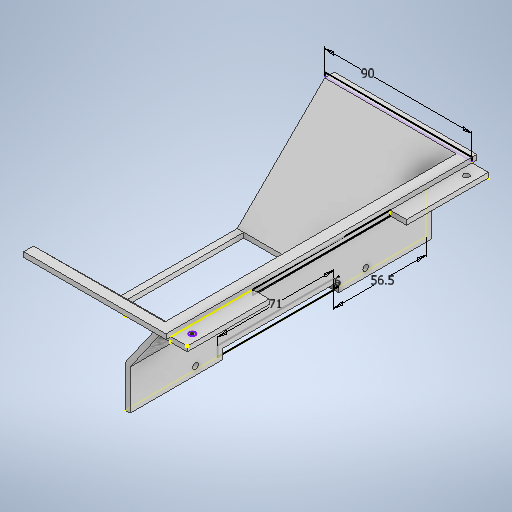
# Autodesk Inventor part: D2-CA
Saved by Autodesk Inventor 2025.2 (Build 292293000, 293)
## iProperties
Created: 2025-11-16
Part Number: D2-CA
Material: 일반
Document SubType Name: Modeling
Designer: RunGeun
Density: 1 g/cm^3
Appearance: 기본값
Author: RunGeun
Autodesk Inventor part; units mm, degrees
ref_plane "YZ Plane" through (0, 0, 0) normal (1, 0, 0) x (0, 1, 0)
ref_plane "XZ Plane" through (0, 0, 0) normal (0, 1, 0) x (-1, 0, 0)
ref_plane "XY Plane" through (0, 0, 0) normal (0, 0, 1) x (1, 0, 0)
sketch "스케치1" plane through (0, 0, 0) normal (0, 1, 0) x (-1, 0, 0)
  line L0 (0, 0) -> (10, 0)
  line L1 (10, 0) -> (10, -184)
  line L2 (10, -184) -> (0, -184)
  line L3 (0, -184) -> (0, 0)
  circle A0 centre (5, -175.5766) radius 1.75
  circle A1 centre (5, -8.1019) radius 1.75
  dimension "d0" = 184
  dimension "d1" = 10
  dimension "d2" = 5
  dimension "d3" = 3.5
  dimension "d4" = 3.5
  dimension "d5" = 5
  dimension "d109" = 167.4748
  constraints: 8 end point, 2 centre point, 2 parallel, 1 horizontal, 1 perpendicular
  measures "d0" distance of L2.end L0.start
  measures "d1" distance of L1.end L2.end
  measures "d2" distance from line of A0.centre L1
  measures "d3" diameter of A0
  measures "d4" diameter of A1
  measures "d5" distance from line of A1.centre L1
  measures "d109" distance of A0.centre A1.centre
extrude "돌출1" add sketch "스케치1" along normal blind 3
sketch "스케치2" plane through (-10, 0, -184) normal (-1, 0, 0) x (0, 0, 1)
  line L0 (187, 0) -> (-3, 0)
  line L1 (-3, 0) -> (-3, 6)
  line L2 (-3, 6) -> (187, 6)
  line L3 (187, 6) -> (187, 0)
  line L4 (0, 0) -> (0, 3) projected
  line L5 (184, 0) -> (184, 3) projected
  line L6 (0, 3) -> (184, 3) projected
  line L7 (187, 0) -> (-3, 0)
  line L8 (-3, 0) -> (-3, 3)
  line L9 (-3, 3) -> (187, 3)
  line L10 (187, 3) -> (187, 0)
  dimension "d8" = 3
  dimension "d9" = 3
  dimension "d10" = 3
  constraints: 16 end point, 4 parallel, 2 horizontal, 2 perpendicular, 1 midpoint
  measures "d8" distance between parallel lines of L4 L1
  measures "d9" distance between parallel lines of L5 L3
  measures "d10" distance between parallel lines of L6 L2
extrude "돌출2" add sketch "스케치2" along normal blind 3 contours L0 L4 L6 L5 | L9 L6 L1 L2 L3
sketch "스케치3" plane through (-10, 3, -187) normal (0, 0, -1) x (-1, 0, 0)
  line L0 (0, 3) -> (3, 3) projected
  line L1 (0, 3) -> (28, 3)
  line L2 (28, 3) -> (28, -48)
  line L3 (28, -48) -> (0, -48)
  line L4 (0, -48) -> (0, 3)
  line L5 (3, 3) -> (25, -28.5697)
  line L6 (25, -28.5697) -> (25, -48)
  line L7 (6.6566, 3) -> (28, -27.6275)
  line L8 (3, 0) -> (3, -3) projected
  line L9 (3, -3) -> (7.1812, -3)
  line L10 (3, -3) -> (6.6592, -3)
  line L11 (6.6592, -3) -> (6.6592, 3)
  line L12 (6.6592, 3) -> (3, 3)
  line L13 (3, 3) -> (3, -3)
  line L14 (28, -48) -> (25, -48)
  line L15 (25, -48) -> (25, -53)
  line L16 (25, -53) -> (28, -53)
  line L17 (28, -53) -> (28, -48)
  point P0 (-10, -3)
  dimension "d14" = 51
  dimension "d15" = 28
  dimension "d18" = 5
  dimension "d31" = 3
  dimension "d32" = 3
  dimension "d33" = 3
  constraints: 32 end point, 7 parallel, 5 perpendicular, 5 point on line, 3 horizontal
  measures "d14" distance of L1.end L2.end
  measures "d15" distance of L0.start L1.end
  measures "d18" distance of L15.end L14.end
  measures "d31" distance of L15.end L16.end
  measures "d32" distance between parallel lines of L2 L6
  measures "d33" distance between parallel lines of L7 L5
extrude "돌출3" add sketch "스케치3" against normal blind 190 contours L1 L7 L11 L5 | L5 L11 L9 L8 L13 | L11 L7 L2 L3 L6 L5 | L5 L9 L11 | L3 L17 L16 L15
sketch "스케치4" plane through (-10, 3, -187) normal (0, 0, -1) x (-1, 0, 0)
  line L0 (28, -53) -> (25, -53) projected
  line L1 (3, 0) -> (3, -3) projected
  line L2 (28, -53) -> (3, -53)
  line L3 (3, -53) -> (3, 0)
  line L4 (3, 0) -> (28, 0)
  line L5 (28, 0) -> (28, -53)
  point P0 (-10, -3)
  constraints: 8 end point, 2 parallel, 1 horizontal, 1 perpendicular
extrude "돌출4" cut sketch "스케치4" against normal blind 3
sketch "스케치5" plane through (-10, 3, 3) normal (0, 0, 1) x (1, 0, 0)
  line L0 (-28, -53) -> (-25, -53) projected
  line L1 (-3, -3) -> (-3, 0) projected
  line L2 (-28, -53) -> (-3, -53)
  line L3 (-3, -53) -> (-3, 0)
  line L4 (-3, 0) -> (-28, 0)
  line L5 (-28, 0) -> (-28, -53)
  point P0 (10, -3)
  constraints: 8 end point, 2 parallel, 1 horizontal, 1 perpendicular
extrude "돌출5" cut sketch "스케치5" against normal blind 3
sketch "스케치6" plane through (-38, -50, 0) normal (-1, 0, 0) x (0, 0, 1)
  circle A0 centre (-40, 5) radius 1.75
  circle A1 centre (-144, 5) radius 1.75
  line L0 (-184, 0) -> (0, 0) projected
  line L1 (0, 0) -> (0, 25.3725) projected
  point P0 (0, 50)
  dimension "d23" = 3.5
  dimension "d24" = 3.5
  dimension "d25" = 5
  dimension "d26" = 5
  dimension "d27" = 104
  dimension "d28" = 40
  constraints: 2 centre point
  measures "d23" diameter of A1
  measures "d24" diameter of A0
  measures "d25" distance from line of A1.centre L0
  measures "d26" distance from line of A0.centre L0
  measures "d27" distance of A1.centre A0.centre
  measures "d28" distance from line of A0.centre L1
extrude "돌출6" cut sketch "스케치6" against normal blind 3
sketch "스케치7" plane through (-38, -50, 0) normal (-1, 0, 0) x (0, 0, 1)
  line L0 (-184, 0) -> (0, 0) projected
  line L1 (-56.5, 0) -> (-127.5, 0)
  line L2 (-127.5, 0) -> (-127.5, 6)
  line L3 (-127.5, 6) -> (-56.5, 6)
  line L4 (-56.5, 6) -> (-56.5, 0)
  line L5 (-184, 25.3725) -> (-184, 0) projected
  point P0 (0, 50)
  point P1 (-127.5, 0)
  dimension "d34" = 71
  dimension "d35" = 6
  dimension "d102" = 56.5
  constraints: 8 end point, 2 parallel, 1 horizontal, 1 perpendicular, 1 point on line
  measures "d34" distance of L2.end L3.end
  measures "d35" distance of L1.end L2.end
  measures "d102" distance from line of L5 L2.end
extrude "돌출7" cut sketch "스케치7" against normal blind 3
sketch "스케치8" plane through (-38, -50, 0) normal (-1, 0, 0) x (0, 0, 1)
  line L0 (0, 0) -> (-35, 0)
  line L1 (-35, 0) -> (-35, 3)
  line L2 (-35, 3) -> (0, 3)
  line L3 (0, 3) -> (0, 0)
  line L4 (-184, 0) -> (-184, 24.4303) projected
  line L5 (-184, 0) -> (-149, 0)
  line L6 (-149, 0) -> (-149, 3)
  line L7 (-149, 3) -> (-184, 3)
  line L8 (-184, 3) -> (-184, 0)
  circle A0 centre (-40, 5) radius 1.75 projected
  line L9 (-56.5, 0) -> (-56.5, 6) projected
  line L10 (-56.5, 0) -> (-45, 0)
  line L11 (-45, 0) -> (-45, 3)
  line L12 (-45, 3) -> (-56.5, 3)
  line L13 (-56.5, 3) -> (-56.5, 0)
  circle A1 centre (-144, 5) radius 1.75 projected
  line L14 (-184, 0) -> (-127.5, 0) projected
  line L15 (-127.5, 0) -> (-139, 0)
  line L16 (-139, 0) -> (-139, 3)
  line L17 (-139, 3) -> (-127.5, 3)
  line L18 (-127.5, 3) -> (-127.5, 0)
  line L19 (-139, 0) -> (-149, 0)
  line L20 (-149, 0) -> (-149, 10)
  line L21 (-149, 10) -> (-139, 10)
  line L22 (-139, 10) -> (-139, 0)
  line L23 (-184, 0) -> (-127.5, 0) projected
  line L24 (-136, 0) -> (-152, 0)
  line L25 (-152, 0) -> (-152, 13)
  line L26 (-152, 13) -> (-136, 13)
  line L27 (-136, 13) -> (-136, 0)
  line L28 (-35, 0) -> (-45, 0)
  line L29 (-45, 0) -> (-45, 10)
  line L30 (-45, 10) -> (-35, 10)
  line L31 (-35, 10) -> (-35, 0)
  line L32 (-56.5, 0) -> (0, 0) projected
  line L33 (-32, 0) -> (-48, 0)
  line L34 (-48, 0) -> (-48, 13)
  line L35 (-48, 13) -> (-32, 13)
  line L36 (-32, 13) -> (-32, 0)
  point P0 (0, 50)
  point P1 (-139, 1.5)
  point P2 (-152, 3)
  point P3 (-184, 3)
  point P4 (-149, 3)
  point P5 (-139, 3)
  point P6 (-136, 3)
  point P7 (-32, 3)
  point P8 (-48, 3)
  point P9 (-45, 3)
  point P10 (-35, 3)
  dimension "d38" = 3
  dimension "d39" = 3
  dimension "d41" = 5
  dimension "d42" = 3
  dimension "d43" = 5
  dimension "d44" = 5
  dimension "d45" = 3
  dimension "d46" = 5
  dimension "d47" = 5
  dimension "d48" = 0
  dimension "d49" = 0
  dimension "d50" = 3
  dimension "d51" = 3
  dimension "d52" = 3
  dimension "d53" = 5
  dimension "d54" = 3
  dimension "d55" = 3
  dimension "d56" = 3
  dimension "d57" = 0
  constraints: 64 end point, 16 parallel, 8 horizontal, 8 perpendicular, 3 point on line, 1 midpoint
  measures "d38" distance of L5.end L6.end
  measures "d39" distance between parallel lines of L0 L2
  measures "d41" distance from line of A0.centre L1
  measures "d42" distance of L11.end L10.end
  measures "d43" distance from line of A0.centre L11
  measures "d44" distance from line of A1.centre L6
  measures "d45" distance of L15.end L16.end
  measures "d46" distance from line of A1.centre L16
  measures "d47" distance from line of A1.centre L21
  measures "d48" distance between parallel lines of L6 L20
  measures "d49" distance from line of point (-139, 1.5) L22
  measures "d50" distance between parallel lines of L20 L25
  measures "d51" distance between parallel lines of L27 L22
  measures "d52" distance between parallel lines of L26 L21
  measures "d53" distance from line of A0.centre L30
  measures "d54" distance between parallel lines of L29 L34
  measures "d55" distance between parallel lines of L30 L35
  measures "d56" distance between parallel lines of L36 L31
  measures "d57" distance between parallel lines of L29 L11
extrude "돌출8" add sketch "스케치8" along normal blind 55 contours L0 L36 L2 L3 | L0 L1 L2 L36 | L2 L31 L30 L29 L12 L34 L35 L36 | L10 L34 L12 L11 | L10 L9 L12 L34 | L4 L7 L25 L5 | L25 L7 L6 L5 | L25 L26 L27 L17 L22 L21 L20 L7 | L16 L17 L27 L14 | L27 L17 L18 L14
sketch "스케치12" plane through (0, 3, -184) normal (0, 0, -1) x (-1, 0, 0)
  line L0 (10, 3) -> (10, 0) projected
  line L1 (10, 3) -> (100, 3)
  line L2 (100, 3) -> (100, 0.8239)
  line L3 (100, 0.8239) -> (10, 0.8239)
  line L4 (10, 0.8239) -> (10, 3)
  point P0 (0, -3)
  dimension "d87" = 90
  constraints: 8 end point, 2 parallel, 1 horizontal, 1 perpendicular
  measures "d87" distance of L0.start L1.end
sketch "스케치13" plane through (-93, -50, 0) normal (-1, 0, 0) x (0, 0, 1)
  line L0 (0, 3) -> (-32, 3) projected
  line L1 (-184, 0) -> (-184, 24.4303) projected
  line L2 (0, 3) -> (-184, 3)
  line L3 (-184, 3) -> (-184, 0)
  line L4 (-184, 0) -> (0, 0)
  line L5 (0, 0) -> (0, 3)
  line L6 (-32, 3) -> (-32, 13) projected
  line L7 (-48, 3) -> (-48, 13) projected
  line L8 (-32, 13) -> (-48, 13)
  line L9 (-48, 13) -> (-48, 3)
  line L10 (-48, 3) -> (-32, 3)
  line L11 (-32, 3) -> (-32, 13)
  line L12 (-45, 10) -> (-45, 0) projected
  line L13 (-35, 10) -> (-35, 0) projected
  line L14 (-45, 10) -> (-35, 10)
  line L15 (-35, 10) -> (-35, 3)
  line L16 (-35, 3) -> (-45, 3)
  line L17 (-45, 3) -> (-45, 10)
  line L18 (-136, 3) -> (-136, 13) projected
  line L19 (-152, 3) -> (-152, 13) projected
  line L20 (-136, 3) -> (-152, 3)
  line L21 (-152, 3) -> (-152, 13)
  line L22 (-152, 13) -> (-136, 13)
  line L23 (-136, 13) -> (-136, 3)
  line L24 (-149, 10) -> (-149, 0) projected
  line L25 (-139, 10) -> (-139, 0) projected
  line L26 (-149, 10) -> (-139, 10)
  line L27 (-139, 10) -> (-139, 3)
  line L28 (-139, 3) -> (-149, 3)
  line L29 (-149, 3) -> (-149, 10)
  point P0 (0, 50)
  point P1 (-48, 13)
  point P2 (-45, 3)
  point P3 (-35, 3)
  point P4 (-136, 13)
  constraints: 40 end point, 10 parallel, 5 horizontal, 5 perpendicular, 4 point on line
extrude "돌출11" add sketch "스케치13" along normal blind 7 contours L5 L4 L13 L2 L0 | L2 L13 L14 L12 L7 L8 L6 | L13 L4 L12 L2 | L12 L4 L25 L2 | L4 L24 L2 L25 | L2 L25 L26 L24 L19 L22 L18 | L4 L1 L2 L24
sketch "스케치14" plane through (-100, -50, 0) normal (-1, 0, 0) x (0, 0, 1)
  line L0 (-187, 56) -> (3, 56) projected
  line L1 (0, 0) -> (-3, 0)
  line L2 (-3, 0) -> (-3, 56)
  line L3 (-3, 56) -> (0, 56)
  line L4 (0, 56) -> (0, 0)
  line L5 (-56.5, 6) -> (-56.5, 3) projected
  line L6 (-3, 56) -> (-56.5, 3)
  line L7 (-184, 0) -> (-181, 0)
  line L8 (-181, 0) -> (-181, 56)
  line L9 (-181, 56) -> (-184, 56)
  line L10 (-184, 56) -> (-184, 0)
  line L11 (-127.5, 3) -> (-127.5, 6) projected
  line L12 (-181, 56) -> (-127.5, 3)
  line L13 (-3, 49.7958) -> (-5, 49.7958)
  line L14 (-5, 49.7958) -> (-54.1979, 1.0577)
  line L15 (-181, 49.7958) -> (-179, 49.7958)
  line L16 (-179, 49.7958) -> (-131.7627, 3)
  line L17 (-48, 3) -> (-136, 3) projected
  line L18 (0, 53) -> (-184, 53) projected
  line L19 (3, 56) -> (-3, 56)
  line L20 (-3, 56) -> (-3, 53)
  line L21 (-3, 53) -> (3, 53)
  line L22 (3, 53) -> (3, 56)
  line L23 (-181, 56) -> (-187, 56)
  line L24 (-187, 56) -> (-187, 53)
  line L25 (-187, 53) -> (-181, 53)
  line L26 (-181, 53) -> (-181, 56)
  line L27 (-8.9071, 50.1481) -> (-6.7958, 48.0168)
  line L28 (-6.7958, 48.0168) -> (0, 54.7491)
  line L29 (0, 54.7491) -> (-2.1113, 56.8804)
  line L30 (-2.1113, 56.8804) -> (-8.9071, 50.1481)
  line L31 (-174.0172, 49.0825) -> (-176.1285, 46.9512)
  line L32 (-176.1285, 46.9512) -> (-185.3697, 56.106)
  line L33 (-185.3697, 56.106) -> (-183.2583, 58.2372)
  line L34 (-183.2583, 58.2372) -> (-174.0172, 49.0825)
  point P0 (0, 50)
  point P1 (-52.2373, 3)
  point P2 (-182.2344, 53)
  point P3 (-1.7656, 53)
  dimension "d90" = 3
  dimension "d91" = 3
  dimension "d92" = 3
  dimension "d93" = 2
  dimension "d94" = 3
  dimension "d95" = 2
  constraints: 60 end point, 14 parallel, 12 point on line, 9 perpendicular, 5 horizontal
  measures "d90" distance of L2.end L3.end
  measures "d91" distance between parallel lines of L10 L8
  measures "d92" distance between parallel lines of L6 L14
  measures "d93" distance of L13.start L13.end
  measures "d94" distance between parallel lines of L12 L16
  measures "d95" distance of L15.start L15.end
extrude "돌출12" add sketch "스케치14" against normal blind 90 contours L10 L32 L0 | L0 L8 L18 L32 L10 | L12 L18 L8 | L32 L10 L25 L24 L0 | L32 L18 L10 | L0 L29 L28 L18 L2 | L2 L18 L6 | L18 L12 L31 L16 L32 L8 | L8 L32 L18 | L0 L4 L29 | L18 L28 L2 | L2 L28 L14 L27 L6 L18 | L12 L17 L16 L31 | L0 L22 L21 L4 | L4 L18 L28 | L27 L14 L17 L6
sketch "스케치15" plane through (-100, -50, 0) normal (-1, 0, 0) x (0, 0, 1)
  line L0 (44.6892, 116.5237) -> (-211.4065, 116.5237)
  line L1 (-211.4065, 116.5237) -> (-211.4065, -47.1327)
  line L2 (-211.4065, -47.1327) -> (44.6892, -47.1327)
  line L3 (44.6892, -47.1327) -> (44.6892, 116.5237)
  point P0 (0, 50)
  constraints: 8 end point, 2 parallel, 1 horizontal, 1 perpendicular
extrude "돌출13" cut sketch "스케치15" against normal blind 3
sketch "스케치16" plane through (0, 0, -184) normal (0, 0, -1) x (-1, 0, 0)
  line L0 (17.1812, 0) -> (35, -25.5697) projected
  line L1 (17.1812, 0) -> (0, 0)
  line L2 (0, 0) -> (0, -57.2886)
  line L3 (0, -57.2886) -> (17.1812, -57.2886)
  line L4 (17.1812, -57.2886) -> (17.1812, 0)
  line L5 (17.1812, -57.2886) -> (35, -57.2886)
  line L6 (35, -57.2886) -> (35, -25.5697)
  line L7 (35, -25.5697) -> (17.1812, -25.5697)
  line L8 (17.1812, -25.5697) -> (17.1812, -57.2886)
  line L9 (17.1812, 0) -> (35, -25.5697)
  point P0 (0, 0)
  constraints: 18 end point, 5 equal length, 2 horizontal, 2 perpendicular
extrude "돌출14" cut sketch "스케치16" against normal through all
sketch "스케치17" plane through (-97, -50, 0) normal (-1, 0, 0) x (0, 0, 1)
  line L0 (-46.4057, 13) -> (-33.9164, 25.3725) projected
  line L1 (-45.6744, 13.7244) -> (-49.5898, 9.8456)
  line L2 (-49.5898, 9.8456) -> (-52.0162, 12.2948)
  line L3 (-52.0162, 12.2948) -> (-48.1007, 16.1737)
  line L4 (-48.1007, 16.1737) -> (-45.6744, 13.7244)
  line L5 (-150.0836, 25.3725) -> (-137.5943, 13) projected
  line L6 (-138.3256, 13.7244) -> (-134.7016, 10.1343)
  line L7 (-134.7016, 10.1343) -> (-131.5484, 13.3172)
  line L8 (-131.5484, 13.3172) -> (-135.1724, 16.9074)
  line L9 (-135.1724, 16.9074) -> (-138.3256, 13.7244)
  line L10 (-179, 49.7958) -> (-125.2859, -3.4163)
  line L11 (-125.2859, -3.4163) -> (-162.2217, -40.7006)
  line L12 (-162.2217, -40.7006) -> (-215.9358, 12.5116)
  line L13 (-215.9358, 12.5116) -> (-179, 49.7958)
  line L14 (-48, 7.1977) -> (-42.143, 13) projected
  line L15 (-5, 49.7958) -> (-57.5764, -2.2892)
  line L16 (-57.5764, -2.2892) -> (-11.67, -48.6286)
  line L17 (-11.67, -48.6286) -> (40.9064, 3.4564)
  line L18 (40.9064, 3.4564) -> (-5, 49.7958)
  point P0 (0, 50)
  point P1 (-42.143, 13)
  constraints: 32 end point, 8 parallel, 4 perpendicular, 3 collinear, 2 point on line
extrude "돌출15" cut sketch "스케치17" against normal blind 59
sketch "스케치18" plane through (0, 3, 0) normal (0, 1, 0) x (1, 0, 0)
  line L0 (0, 0) -> (0, 184) projected
  line L1 (-10, 184) -> (-10, 0) projected
  line L2 (0, 50) -> (-10, 50)
  line L3 (-10, 50) -> (-10, 134)
  line L4 (-10, 134) -> (0, 134)
  line L5 (0, 134) -> (0, 50)
  line L6 (0, 184) -> (-10, 184) projected
  line L7 (-10, 0) -> (0, 0) projected
  point P0 (-5, 184)
  point P1 (-5, 0)
  point P2 (0, 134)
  dimension "d105" = 50
  dimension "d106" = 50
  constraints: 8 end point, 2 midpoint, 2 parallel, 2 point on line, 1 horizontal, 1 perpendicular
  measures "d105" distance from line of point (-5, 184) L4
  measures "d106" distance from line of point (-5, 0) L2
extrude "돌출16" cut sketch "스케치18" against normal blind 90 contours L2 L1 L4 L0
sketch "스케치19" plane through (-10, 0, -184) normal (1, 0, 0) x (0, 0, -1)
  line L0 (-50, 3) -> (-50, 0) projected
  line L1 (-134, 3) -> (-184, 3) projected
  line L2 (-50, 0) -> (-134, 0)
  line L3 (-134, 0) -> (-134, 3)
  line L4 (-134, 3) -> (-50, 3)
  line L5 (-50, 3) -> (-50, 0)
  point P0 (-184, 0)
  constraints: 8 end point, 2 parallel, 1 horizontal, 1 perpendicular
sketch "스케치20" plane through (0, 3, 0) normal (0, 1, 0) x (1, 0, 0)
  circle A0 centre (-5, 8.1019) radius 1.75 projected
  circle A1 centre (-5, 8.1019) radius 1.75
  point P0 (0, 0)
  constraints: 1 centre point, 1 coincident
equation "\"d4\" = d3"
equation "\"d5\" = d2"
equation "\"d24\" = d23"
equation "\"d26\" = d25"
equation "\"d39\" = d38"
equation "\"d43\" = d41"
equation "\"d44\" = d41"
equation "\"d46\" = d44"
equation "\"d50\" = d52"
equation "\"d51\" = d52"
equation "\"d53\" = d41"
equation "\"d54\" = d52"
equation "\"d55\" = d54"
equation "\"d56\" = d54"
equation "\"d106\" = d105"
